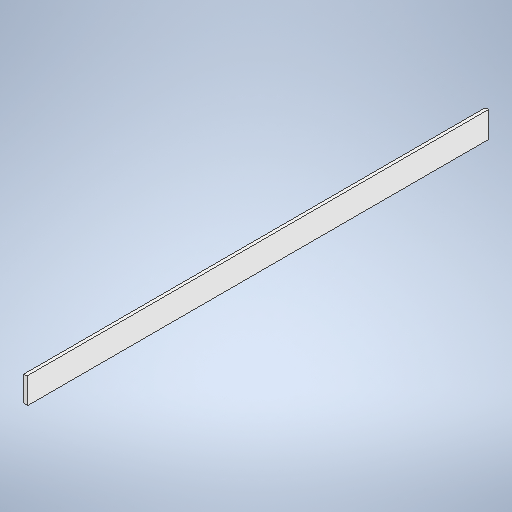
# Autodesk Inventor part: Fascia_For_Back
Saved by Autodesk Inventor 2025 (Build 290162010, 162A)
## iProperties
Created: 2024-09-15
Part Number: Fascia_For_Back
Material: Generic
Document SubType Name: Modeling
Designer: Tom
Density: 1 g/cm^3
Appearance: White
Author: Tom
Autodesk Inventor part; units mm, degrees
ref_plane "YZ Plane" through (0, 0, 0) normal (1, 0, 0) x (0, 1, 0)
ref_plane "XZ Plane" through (0, 0, 0) normal (0, 1, 0) x (-1, 0, 0)
ref_plane "XY Plane" through (0, 0, 0) normal (0, 0, 1) x (1, 0, 0)
sketch "Sketch1" plane through (0, 0, 0) normal (0, 0, 1) x (1, 0, 0)
  line L0 (0, 0) -> (3263.9, 1089.025)
  line L1 (0, 0) -> (-88.9, 0)
  line L2 (25.4, 8.4749) -> (25.4, -131.2251)
  line L3 (25.4, -131.2251) -> (0, -131.2251)
  line L4 (0, -131.2251) -> (0, 0)
  dimension "d33" = 1089.025
  dimension "d36" = 3352.8
  dimension "d37" = 88.9
  dimension "d42" = 25.4
  dimension "d43" = 139.7
  constraints: 10 end point, 2 coincident, 2 perpendicular, 1 horizontal, 1 point on line, 1 vertical
  measures "d33" vertical distance of L0.end point (0, 0)
  measures "d36" horizontal distance of L1.end L0.end
  measures "d37" distance of point (0, 0) L1.end
  measures "d42" distance between parallel lines of L4 L2
  measures "d43" distance of L2.start L2.end
extrude "Extrusion3" add sketch "Sketch1" along normal blind 2476.6016
body "Solid3"
